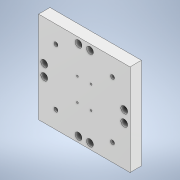
# Autodesk Inventor part: 土台
Saved by Autodesk Inventor 2021 (Build 250183000, 183)
## iProperties
Created: 2021-10-07
Part Number: 土台
Material: 一般
Document SubType Name: Modeling
Designer: ryusei
Density: 1 g/cm^3
Appearance: 滑らか - 白
Author: ryusei
Autodesk Inventor part; units mm, degrees
ref_plane "YZ Plane" through (0, 0, 0) normal (1, 0, 0) x (0, 1, 0)
ref_plane "XZ Plane" through (0, 0, 0) normal (0, 1, 0) x (-1, 0, 0)
ref_plane "XY Plane" through (0, 0, 0) normal (0, 0, 1) x (1, 0, 0)
sketch "スケッチ1" plane through (0, 0, 0) normal (0, 0, 1) x (1, 0, 0)
  line L0 (0, 0) -> (80, 0)
  line L1 (80, 0) -> (80, 80)
  line L2 (80, 80) -> (0, 80)
  line L3 (0, 80) -> (0, 0)
  dimension "d0" = 80
  dimension "d1" = 80
  constraints: 8 end point, 2 parallel, 1 horizontal, 1 perpendicular
  measures "d0" distance between parallel lines of L1 L3
  measures "d1" distance between parallel lines of L0 L2
extrude "押し出し1" add sketch "スケッチ1" along normal blind 10
sketch "スケッチ2" plane through (0, 0, 10) normal (0, 0, 1) x (1, 0, 0)
  line L0 (80, 80) -> (0, 80) projected
  line L1 (80, 0) -> (80, 80) projected
  line L2 (0, 0) -> (80, 0) projected
  line L3 (40, 80) -> (40, 0)
  point P0 (45, 75)
  point P1 (75, 45)
  point P2 (75, 35)
  point P3 (45, 5)
  point P4 (35, 75)
  point P5 (5, 45)
  point P6 (5, 35)
  point P7 (35, 5)
  dimension "d4" = 5
  dimension "d5" = 5
  dimension "d6" = 5
  dimension "d7" = 5
  dimension "d8" = 35
  dimension "d9" = 35
  dimension "d10" = 35
  dimension "d11" = 35
  constraints: 4 symmetric about line, 2 end point, 2 midpoint
  measures "d4" distance from line of L0 point (45, 75)
  measures "d5" distance from line of L1 point (75, 45)
  measures "d6" distance from line of L1 point (75, 35)
  measures "d7" distance from line of L2 point (45, 5)
  measures "d8" distance from line of L2 point (75, 35)
  measures "d9" distance from line of L1 point (45, 5)
  measures "d10" distance from line of L0 point (75, 45)
  measures "d11" distance from line of point (45, 75) L1
hole "穴1" at (45, 75, 10) at (75, 45, 10) at (75, 35, 10) at (45, 5, 10) at (35, 75, 10) at (5, 45, 10) at (5, 35, 10) at (35, 5, 10) direction (0, 0, -1) diameter 3.5 end through all counterbore diameter 6 counterbore depth 4
sketch "スケッチ10" plane through (0, 0, 10) normal (0, 0, 1) x (1, 0, 0)
  line L0 (0, 80) -> (0, 0) projected
  line L1 (80, 80) -> (0, 80) projected
  line L2 (0, 0) -> (80, 80)
  line L3 (80, 0) -> (80, 80) projected
  line L4 (80, 0) -> (0, 80)
  point P0 (15.2513, 64.7487)
  point P1 (64.7487, 15.2513)
  point P2 (15.2513, 15.2513)
  point P3 (64.7487, 64.7487)
  dimension "d41" = 70
  dimension "d42" = 70
  constraints: 4 end point, 2 point on line, 2 symmetric about line
  measures "d41" diameter of point (15.251, 64.749) L2
  measures "d42" diameter of point (15.251, 15.251) L4
hole "穴3" at (15.2513, 64.7487, 10) at (64.7487, 15.2513, 10) at (15.2513, 15.2513, 10) at (64.7487, 64.7487, 10) direction (0, 0, -1) diameter 3.5 end through all
sketch "スケッチ12" plane through (0, 0, 10) normal (0, 0, 1) x (1, 0, 0)
  line L0 (0, 80) -> (0, 0) projected
  line L1 (0, 40) -> (80, 40)
  line L2 (80, 0) -> (80, 80) projected
  line L3 (80, 80) -> (0, 80) projected
  line L4 (40, 80) -> (40, 0)
  line L5 (0, 0) -> (80, 0) projected
  line L6 (40, 60) -> (40, -20)
  line L7 (52, 80) -> (52, 0)
  line L8 (52, 60) -> (52, -20)
  point P0 (34, 50)
  point P1 (34, 30)
  point P2 (46, 50)
  point P3 (46, 30)
  dimension "d68" = 12
  dimension "d69" = 20
  dimension "d72" = 20
  dimension "d75" = 12
  constraints: 10 end point, 4 midpoint, 1 collinear, 1 horizontal, 1 vertical, 11 other
  measures "d68" diameter of point (34, 50) L4
  measures "d69" diameter of point (34, 50) L1
  measures "d72" distance of point (34, 50) point (34, 30)
  measures "d75" distance of point (34, 50) point (46, 50)
hole "穴5" at (34, 50, 10) at (34, 30, 10) at (46, 50, 10) at (46, 30, 10) direction (0, 0, -1) diameter 1.567 end through all thread size "M2x0.4" class "6H" standard "ISO Metric profile"
